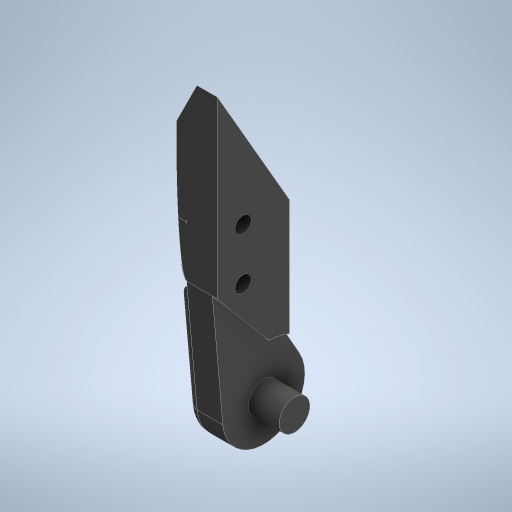
# Autodesk Inventor part: side_left
Saved by Autodesk Inventor 2024.1 (Build 281209000, 209)
## iProperties
Created: 2024-10-11
Part Number: side_left
Material: 一般
Document SubType Name: Modeling
Designer: hibik
Density: 1 g/cm^3
Appearance: 既定
Author: hibik
Autodesk Inventor part; units mm, degrees
ref_plane "YZ Plane" through (0, 0, 0) normal (1, 0, 0) x (0, 1, 0)
ref_plane "XZ Plane" through (0, 0, 0) normal (0, 1, 0) x (-1, 0, 0)
ref_plane "XY Plane" through (0, 0, 0) normal (0, 0, 1) x (1, 0, 0)
sketch "スケッチ1" plane through (0, 0, 0) normal (1, 0, 0) x (0, 1, 0)
  line L0 (0, 0) -> (50, 0)
  line L1 (50, 0) -> (50, -7)
  line L2 (50, -7) -> (0, -7)
  line L3 (0, -7) -> (0, 0)
  line L4 (50, 0) -> (37.8756, -7)
  dimension "d0" = 7
  dimension "d1" = 120
  dimension "d2" = 50
  constraints: 10 end point, 2 parallel, 1 horizontal, 1 perpendicular, 1 point on line
  measures "d0" distance of L0.end L1.end
  measures "d1" angle of L1 L4
  measures "d2" distance of L1.end L2.end
extrude "押し出し1" add sketch "スケッチ1" along normal blind 4 contours L0 L4 L2 L3
sketch "スケッチ2" plane through (0, 0, 0) normal (-1, 0, 0) x (0, 0, 1)
  arc A0 (-5.0347, 26.9903) -> (-7, 26.573) centre (-5, 21.9904) ccw projected
  circle A1 centre (-5, 21.9904) radius 1.5
  circle A2 centre (-5, 21.9904) radius 4
  line L0 (-7, 26.573) -> (-8.4796, 23.9632)
  line L1 (0, 32.9904) -> (-5.0347, 26.9903) projected
  line L2 (0, 32.9904) -> (-1.0159, 21.634)
  line L3 (0, 0) -> (-7, 0) projected
  line L4 (0, 50) -> (0, 0) projected
  line L5 (-7, 37.8756) -> (0, 50) projected
  line L6 (-7, 0) -> (-7, 37.8756) projected
  point P0 (-7, 18.5263)
  dimension "d5" = 3
  dimension "d6" = 8
  constraints: 4 end point, 2 centre point, 2 coincident, 2 point on circle, 2 tangent
  measures "d5" diameter of A1
  measures "d6" diameter of A2
extrude "押し出し2" cut sketch "スケッチ2" against normal through all contours L4 L3 L6 A2 L2
sketch "スケッチ3" plane through (0, 0, 0) normal (-1, 0, 0) x (0, 0, 1)
  arc A0 (-7, 18.5263) -> (-1.0159, 21.634) centre (-5, 21.9904) ccw projected
  circle A1 centre (-5, 21.9904) radius 4
  arc A2 (-5.0347, 26.9903) -> (-7, 26.573) centre (-5, 21.9904) ccw projected
  line L0 (-7, 26.573) -> (-8.4796, 23.9632)
  arc A3 (-7, 18.5263) -> (-1.0159, 21.634) centre (-5, 21.9904) ccw projected
  line L1 (-1.0159, 21.634) -> (0, 32.9904) projected
  line L2 (0, 50) -> (0, 32.9904) projected
  line L3 (-7, 37.8756) -> (0, 50) projected
  line L4 (-7, 18.5263) -> (-7, 37.8756) projected
  point P0 (0, 0)
  point P1 (-7, 26.573)
  constraints: 2 end point, 1 coincident, 5 other
extrude "押し出し3" add sketch "スケッチ3" against normal up to surface (4 mm away) contours A1 L4 | L0 L4 A1
sketch "スケッチ4" plane through (0, 0, 0) normal (-1, 0, 0) x (0, 0, 1)
  arc A0 (-5.0347, 26.9903) -> (-7, 26.573) centre (-5, 21.9904) ccw projected
  line L0 (-5.0347, 26.9903) -> (0, 32.9904) projected
  line L1 (0, 32.9904) -> (0, 50) projected
  line L2 (0, 50) -> (7.5, 62.9904) projected
  line L3 (7.5, 62.9904) -> (15, 62.9904) projected
  line L4 (15, 116.9904) -> (15, 62.9904) projected
  line L5 (-7, 116.9904) -> (15, 116.9904) projected
  line L6 (-7, 116.9904) -> (-7, 26.573) projected
  line L7 (13, 104.3691) -> (13, 98.6117) projected
  arc A1 (12.5607, 97.551) -> (13, 98.6117) centre (11.5, 98.6117) ccw projected
  line L8 (12.5607, 97.551) -> (-0.9393, 84.051) projected
  arc A2 (-3.5, 85.1117) -> (-0.9393, 84.051) centre (-2, 85.1117) ccw projected
  line L9 (-3.5, 85.1117) -> (-3.5, 90.8691) projected
  arc A3 (-3.0607, 91.9297) -> (-3.5, 90.8691) centre (-2, 90.8691) ccw projected
  line L10 (-3.0607, 91.9297) -> (10.4393, 105.4297) projected
  arc A4 (13, 104.3691) -> (10.4393, 105.4297) centre (11.5, 104.3691) ccw projected
  line L11 (13, 84.3691) -> (13, 78.6117) projected
  arc A5 (12.5607, 77.551) -> (13, 78.6117) centre (11.5, 78.6117) ccw projected
  line L12 (12.5607, 77.551) -> (-0.9393, 64.051) projected
  arc A6 (-3.5, 65.1117) -> (-0.9393, 64.051) centre (-2, 65.1117) ccw projected
  line L13 (-3.5, 65.1117) -> (-3.5, 70.8691) projected
  arc A7 (-3.0607, 71.9297) -> (-3.5, 70.8691) centre (-2, 70.8691) ccw projected
  line L14 (-3.0607, 71.9297) -> (10.4393, 85.4297) projected
  arc A8 (13, 84.3691) -> (10.4393, 85.4297) centre (11.5, 84.3691) ccw projected
  arc A9 (-8.4796, 23.9632) -> (-1.0159, 21.634) centre (-5, 21.9904) ccw projected
  line L15 (-1.0159, 21.634) -> (0, 32.9904) projected
  line L16 (0, 50) -> (0, 32.9904) projected
  line L17 (-7, 37.8756) -> (0, 50) projected
  line L18 (-7, 26.573) -> (-7, 37.8756) projected
  line L19 (-7, 26.573) -> (-8.4796, 23.9632) projected
  circle A10 centre (-2.5, 37.9904) radius 0.8 projected
  circle A11 centre (-2.5, 32.9904) radius 0.8 projected
  point P0 (0, 0)
  point P1 (-7, 26.573)
extrude "押し出し4" cut sketch "スケッチ4" against normal blind 0.5 contours L0 L15 A9 L19 A0
sketch "スケッチ5" plane through (0.5, 0, 0) normal (-1, 0, 0) x (0, 0, 1)
  arc A0 (-8.4796, 23.9632) -> (-1.0159, 21.634) centre (-5, 21.9904) ccw projected
  circle A1 centre (-5, 21.9904) radius 1.5
  point P0 (0, 0)
  dimension "d13" = 3
  constraints: 1 centre point, 1 coincident
  measures "d13" diameter of A1
extrude "押し出し5" add sketch "スケッチ5" along normal blind 3
chamfer "面取り1" distance 2 angle 45 2 edges at (4, 43.9378, -3.5) (4, 32.2243, -7)
fillet "フィレット1" radius 1 4 edges at (4, 25.2681, -7.7398) (4, 20.94, -8.8596) (4, 18.4405, -3.1565) (4, 27.3122, -0.508)
sketch "スケッチ6" plane through (4, 0, 0) normal (1, 0, 0) x (0, 0, -1)
  circle A0 centre (2.5, 37.9904) radius 0.8
  circle A1 centre (2.5, 32.9904) radius 0.8
  line L0 (0, 32.9904) -> (0, 44.2136) projected
  point P0 (0, 0)
  dimension "d20" = 1.6
  dimension "d21" = 1.6
  dimension "d22" = 2.5
  dimension "d23" = 5
  constraints: 2 centre point, 1 horizontal alignment, 1 vertical alignment
  measures "d20" diameter of A0
  measures "d21" diameter of A1
  measures "d22" distance from line of A0.centre L0
  measures "d23" distance of A0.centre A1.centre
extrude "押し出し6" cut sketch "スケッチ6" against normal through all
sketch "スケッチ7" plane through (4, 0, 0) normal (1, 0, 0) x (0, 0, -1)
  circle A0 centre (2.5, 37.9904) radius 0.8 projected
  circle A1 centre (2.5, 32.9904) radius 0.8 projected
  circle A2 centre (2.5, 37.9904) radius 2.5
  circle A3 centre (2.5, 32.9904) radius 2.5
  point P0 (0, 0)
  point P1 (2.5, 35.4904)
  dimension "d26" = 5
  dimension "d27" = 5
  constraints: 2 centre point, 2 coincident
  measures "d26" diameter of A2
  measures "d27" diameter of A3
extrude "押し出し7" cut sketch "スケッチ7" against normal blind 1 contours A0 | A1 | A2 | A3
mirror "ミラー1" about plane through (0, 25, -3.5) normal (-1, 0, 0) remove original yes
